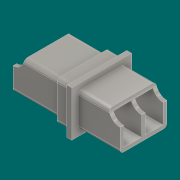
# Autodesk Inventor part: lcLcCoupler
Saved by Autodesk Inventor 2016 SP1 (Build 200210100, 210)
## iProperties
Created: 2016-04-01
Part Number: lcLcCoupler
Material: Stainless Steel
Document SubType Name: Modeling
Designer: sawai
Density: 8 g/cm^3
Appearance: Semi-Polished
Title: Molex 1061152100_sd
Author: sawai
Comments: http://www.molex.com/pdm_docs/sd/1061152100_sd.pdf
Autodesk Inventor part; units mm, degrees
ref_plane "YZ Plane" through (0, 0, 0) normal (1, 0, 0) x (0, 1, 0)
ref_plane "XZ Plane" through (0, 0, 0) normal (0, 1, 0) x (-1, 0, 0)
ref_plane "XY Plane" through (0, 0, 0) normal (0, 0, 1) x (1, 0, 0)
sketch "Sketch1" plane through (0, 0, 0) normal (0, 1, 0) x (-1, 0, 0)
  line L0 (-8.185, 14.605) -> (8.185, 14.605)
  line L1 (8.185, 14.605) -> (8.185, -14.605)
  line L2 (8.185, -14.605) -> (-8.185, -14.605)
  line L3 (-8.185, -14.605) -> (-8.185, 14.605)
  line L4 (-8.185, 14.605) -> (8.185, -14.605) construction
  line L5 (8.185, 14.605) -> (-8.185, -14.605) construction
  point P0 (0, 0)
  dimension "d0" = 16.37
  dimension "d1" = 29.21
  constraints: 12 end point, 2 midpoint, 2 parallel, 1 horizontal, 1 perpendicular
  measures "d0" distance of L1.end L2.end
  measures "d1" distance of L0.end L1.end
extrude "Extrusion1" add sketch "Sketch1" along normal blind 12.4
sketch "Sketch2" plane through (-8.185, 0, 14.605) normal (0, 0, 1) x (1, 0, 0)
  line L0 (16.37, 0) -> (0, 0) projected
  line L1 (16.37, 0) -> (16.37, 12.4) projected
  line L2 (0, 12.4) -> (16.37, 12.4) projected
  line L3 (0, 0) -> (0, 12.4) projected
  line L4 (0, 12.4) -> (16.37, 12.4) projected
  line L5 (16.37, 12.4) -> (0, 0) construction
  line L6 (0, 12.4) -> (16.37, 0) construction
  line L7 (1.785, 1.55) -> (14.585, 1.55)
  line L8 (14.585, 1.55) -> (14.585, 10.85)
  line L9 (14.585, 10.85) -> (1.785, 10.85)
  line L10 (1.785, 10.85) -> (1.785, 1.55)
  line L11 (1.785, 1.55) -> (14.585, 10.85) construction
  line L12 (14.585, 1.55) -> (1.785, 10.85) construction
  point P0 (8.185, 0)
  point P1 (8.185, 6.2)
  dimension "d4" = 12.8
  dimension "d5" = 9.3
  constraints: 16 end point, 3 midpoint, 2 parallel, 1 horizontal, 1 perpendicular
  measures "d4" distance of L9.end L8.end
  measures "d5" distance of L8.end L7.end
extrude "Extrusion2" cut sketch "Sketch2" against normal blind 11.41
sketch "Sketch3" plane through (8.185, 0, -14.605) normal (0, 0, -1) x (-1, 0, 0)
  line L0 (16.37, 0) -> (0, 0) projected
  line L1 (16.37, 0) -> (16.37, 12.4) projected
  line L2 (0, 12.4) -> (16.37, 12.4) projected
  line L3 (0, 0) -> (0, 12.4) projected
  line L4 (1.785, 10.85) -> (14.585, 10.85) projected
  line L5 (1.785, 1.55) -> (1.785, 10.85) projected
  line L6 (14.585, 1.55) -> (1.785, 1.55) projected
  line L7 (14.585, 10.85) -> (14.585, 1.55) projected
  line L8 (15.335, 11.6) -> (1.035, 11.6)
  line L9 (1.035, 11.6) -> (1.035, 0.8)
  line L10 (1.035, 0.8) -> (15.335, 0.8)
  line L11 (15.335, 0.8) -> (15.335, 11.6)
  point P0 (8.185, 0)
  dimension "d8" = 10.8
  constraints: 8 end point, 3 other
  measures "d8" distance between parallel lines of L10 L8
extrude "Extrusion3" cut sketch "Sketch3" against normal blind 16.46 contours L0 L3 L2 L1
sketch "Sketch4" plane through (7.15, 0.8, -14.605) normal (0, 0, -1) x (-1, 0, 0)
  line L0 (0.75, 10.05) -> (13.55, 10.05) projected
  line L1 (13.55, 10.05) -> (13.55, 0.75) projected
  line L2 (13.55, 0.75) -> (0.75, 0.75) projected
  line L3 (0.75, 0.75) -> (0.75, 10.05) projected
  line L4 (0, 10.8) -> (0, 0) projected
  line L5 (0, 0) -> (14.3, 0) projected
  line L6 (14.3, 0) -> (14.3, 10.8) projected
  line L7 (14.3, 10.8) -> (0, 10.8) projected
  point P0 (7.15, -0.8)
extrude "Extrusion4" cut sketch "Sketch4" against normal blind 12.75
sketch "Sketch5" plane through (6.4, 1.55, -14.605) normal (1, 0, 0) x (0, 0, -1)
  line L0 (-29.21, 0) -> (-29.21, 9.3) projected
  line L1 (-29.21, 0) -> (-17.8, 0) projected
  line L2 (-17.8, 0) -> (-17.8, 9.3) projected
  line L3 (-29.21, 9.3) -> (-17.8, 9.3) projected
  line L4 (0, 9.3) -> (0, 0) projected
  line L5 (0, 9.3) -> (-12.75, 9.3) projected
  line L6 (-12.75, 9.3) -> (-12.75, 0) projected
  line L7 (0, 0) -> (-12.75, 0) projected
  circle A0 centre (-29.21, 9.3) radius 3
  line L8 (0, 0) -> (0, 9.3) projected
  circle A1 centre (0, 9.3) radius 3
  point P0 (-14.605, -1.55)
  dimension "d13" = 6
  dimension "d14" = 6
  constraints: 2 centre point, 2 coincident
  measures "d13" diameter of A0
  measures "d14" diameter of A1
extrude "Extrusion5" cut sketch "Sketch5" against normal through all contours A0 L3 L0 | L0 L3 A0 | L5 A1 L4 | L4 A1 L5
sketch "Sketch6" plane through (6.4, 1.55, -14.605) normal (0, 0, -1) x (-1, 0, 0)
  line L0 (0, 9.3) -> (12.8, 9.3) projected
  line L1 (0, 6.3) -> (0, 9.3) projected
  line L2 (0, 6.3) -> (0, 0) projected
  line L3 (12.8, 0) -> (12.8, 6.3) projected
  line L4 (12.8, 9.3) -> (12.8, 6.3) projected
  line L5 (0, 0) -> (12.8, 0) projected
  line L6 (11.8, 8.3) -> (1, 8.3)
  line L7 (1, 8.3) -> (1, 6.3)
  line L8 (1, 6.3) -> (1, 1)
  line L9 (1, 1) -> (11.8, 1)
  line L10 (11.8, 1) -> (11.8, 6.3)
  line L11 (11.8, 6.3) -> (11.8, 8.3)
  line L12 (1, 8.3) -> (11.8, 1) construction
  line L13 (1, 1) -> (11.8, 8.3) construction
  line L14 (5.9, 1) -> (6.9, 1)
  line L15 (6.9, 1) -> (6.9, 8.3)
  line L16 (6.9, 8.3) -> (5.9, 8.3)
  line L17 (5.9, 8.3) -> (5.9, 1)
  line L18 (5.9, 1) -> (6.9, 8.3) construction
  line L19 (6.9, 1) -> (5.9, 8.3) construction
  point P0 (6.4, -1.55)
  point P1 (6.4, 4.65)
  dimension "d17" = 1
  dimension "d18" = 1
  constraints: 28 end point, 3 midpoint, 2 parallel, 1 horizontal, 1 perpendicular, 1 point on line, 5 other
  measures "d17" distance between parallel lines of L0 L6
  measures "d18" distance of L16.end L15.end
extrude "Extrusion6" cut sketch "Sketch6" against normal through all contours L11 L10 L9 L15 L6 | L17 L9 L8 L7 L6
fillet "Fillet1" radius 1 12 edges at (7.15, 11.6, 0) (6.4, 10.85, -6.73) (-7.15, 11.6, 0) (-6.4, 10.85, -6.73) (6.4, 10.85, 7.4) (6.4, 1.55, 8.9) (6.4, 1.55, -8.23) (-6.4, 1.55, -8.23) (-7.15, 0.8, 0) (7.15, 0.8, 0) (-6.4, 1.55, 8.9) (-6.4, 10.85, 7.4)
body "Solid1"
